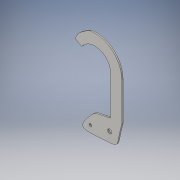
# Autodesk Inventor part: Climb HOok pt 1
Saved by Autodesk Inventor 2016 SP2 (Build 200236200, 236)
## iProperties
Created: 2018-02-07
Part Number: Climb HOok pt 1
Material: Generic
Document SubType Name: Modeling
Designer: CAD
Density: 1 g/cm^3
Appearance: Default
Author: CAD
Autodesk Inventor part; units mm, degrees
ref_plane "YZ Plane" through (0, 0, 0) normal (1, 0, 0) x (0, 1, 0)
ref_plane "XZ Plane" through (0, 0, 0) normal (0, 1, 0) x (-1, 0, 0)
ref_plane "XY Plane" through (0, 0, 0) normal (0, 0, 1) x (1, 0, 0)
sketch "Sketch1" plane through (0, 0, 0) normal (0, 0, 1) x (1, 0, 0)
  line L0 (0, 0) -> (0, 88.9)
  arc A0 (0, 88.9) -> (-43.2611, 124.3295) centre (-36.1384, 88.9) ccw
  arc A1 (25.4, 88.9) -> (-48.2673, 149.2313) centre (-36.1384, 88.9) ccw
  line L1 (25.4, 88.9) -> (25.4, 0)
  line L2 (-48.2673, 149.2313) -> (-79.1061, 132.9539) construction
  line L3 (-79.1061, 132.9539) -> (-80.4219, 116.8588) construction
  spline S0 degree 2 poles (-48.2673, 149.2313) (-79.1061, 132.9539) (-80.4219, 116.8588) knots 1 1 1 2 2 2
  line L4 (-80.4219, 116.8588) -> (-66.3336, 108.7553)
  arc A2 (-43.2611, 124.3295) -> (-66.3336, 108.7553) centre (-36.1384, 88.9) ccw
  spline S1 degree 4 poles (25.4, 0) (6.7382, -69.5402) (37.5135, -31.4962) (-135.4701, -89.9886) (-17.3215, 6.2019) (-45.9643, -12.3049) (0, 0) knots 0 0 0 0 0 0.457859 0.613197 1 1 1 1 1
  point P0 (8.6177, -48.8789)
  point P1 (-30.2905, -52.2043)
  point P2 (-63.6867, -47.8812)
  point P3 (-50.9086, -23.938)
  point P4 (-36.1384, -9.3062)
  dimension "d0" = 88.9
  dimension "d2" = 25.4
  constraints: 7 point on circle, 6 end point, 3 centre point, 1 tangent, 1 vertical, 11 other
  measures "d0" distance of L0.start L0.end
  measures "d2" radial gap between concentric circles of A0 A1
extrude "Extrusion1" add sketch "Sketch1" along normal blind 3.175
sketch "Sketch2" plane through (0, 0, 3.175) normal (0, 0, 1) x (1, 0, 0)
  circle A0 centre (-1.9252, -27.6338) radius 4.7625
  circle A1 centre (-46.0473, -37.5066) radius 3.175
  point P0 (0, 0)
  dimension "d5" = 9.525
  dimension "d6" = 6.35
  constraints: 2 centre point
  measures "d5" diameter of A0
  measures "d6" diameter of A1
extrude "Extrusion2" cut sketch "Sketch2" against normal blind 3.175
body "Solid1"
